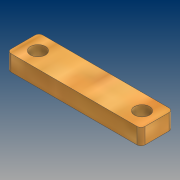
# Autodesk Inventor part: 07_Mieng_go_bu_67x16
Saved by Autodesk Inventor 2021 (Build 250183000, 183)
## iProperties
Created: 2024-04-01
Part Number: 07_Mieng_go_bu_67x16
Material: Laminated Veneer Lumber
Document SubType Name: Modeling
Designer: Admin
Density: 0.51 g/cm^3
Appearance: Plywood - New
Author: Admin
Autodesk Inventor part; units mm, degrees
ref_plane "YZ Plane" through (0, 0, 0) normal (1, 0, 0) x (0, 1, 0)
ref_plane "XZ Plane" through (0, 0, 0) normal (0, 1, 0) x (-1, 0, 0)
ref_plane "XY Plane" through (0, 0, 0) normal (0, 0, 1) x (1, 0, 0)
sketch "Sketch1" plane through (0, 0, 0) normal (0, 1, 0) x (-1, 0, 0)
  line L0 (-33.5, 8) -> (33.5, 8)
  line L1 (33.5, 8) -> (33.5, -8)
  line L2 (33.5, -8) -> (-33.5, -8)
  line L3 (-33.5, -8) -> (-33.5, 8)
  line L4 (-33.5, 8) -> (33.5, -8) construction
  line L5 (33.5, 8) -> (-33.5, -8) construction
  line L6 (46.9, 0) -> (-46.9, 0) construction
  line L7 (0, -11.2) -> (0, 11.2) construction
  line L8 (26, 0) -> (-26, 0)
  circle A0 centre (26, 0) radius 3.75
  circle A1 centre (-26, 0) radius 3.75
  point P0 (0, 0)
  dimension "d0" = 16
  dimension "d1" = 67
  dimension "d2" = 52
  dimension "d3" = 7.5
  constraints: 14 end point, 2 centre point, 2 coincident, 2 midpoint, 2 parallel, 2 point on line, 1 equal radius, 1 horizontal, 1 perpendicular, 1 symmetric about line
  measures "d0" distance of L0.end L1.end
  measures "d1" distance of L1.end L2.end
  measures "d2" distance of L8.end L8.start
  measures "d3" diameter of A0
extrude "Extrusion1" add sketch "Sketch1" along normal blind 8
fillet "Fillet1" radius 2 4 edges at (33.5, 4, 8) (-33.5, 4, 8) (-33.5, 4, -8) (33.5, 4, -8)
body "Solid1"
